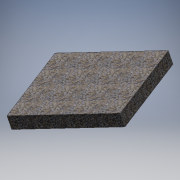
# Autodesk Inventor part: BaseMini
Saved by Autodesk Inventor 2016 (Build 200138000, 138)
## iProperties
Created: 2015-08-01
Part Number: BaseMini
Material: Concrete
Document SubType Name: Modeling
Designer: myhome
Density: 2.40731 g/cm^3
Appearance: Exposed Aggregate - Coarse
Mass: 134809 g
Surface Area: 14200 cm^2
Volume: 56000 cm^3
Author: myhome
Autodesk Inventor part; units mm, degrees
ref_plane "YZ Plane" through (0, 0, 0) normal (1, 0, 0) x (0, 1, 0)
ref_plane "XZ Plane" through (0, 0, 0) normal (0, 1, 0) x (-1, 0, 0)
ref_plane "XY Plane" through (0, 0, 0) normal (0, 0, 1) x (1, 0, 0)
sketch "Sketch5" plane through (0, 0, 0) normal (0, 0, 1) x (1, 0, 0)
  line L0 (0, 0) -> (800, 0)
  line L1 (800, 0) -> (800, 700)
  line L2 (800, 700) -> (0, 700)
  line L3 (0, 700) -> (0, 0)
  dimension "d12" = 800
  dimension "d13" = 700
  constraints: 8 end point, 2 parallel, 1 horizontal, 1 perpendicular
  measures "d12" distance of L1.end L2.end
  measures "d13" distance of L0.end L1.end
extrude "Extrusion4" add sketch "Sketch5" against normal blind 100
body "Solid2"
